Autodesk Inventor part; units mm, degrees
(part 10 of 16)
  spline S60 degree 3 poles (-53.3395, 81.2156) (-53.1853, 81.2213) (-53.0309, 81.2199) (-52.8769, 81.21) (-52.8312, 81.2071) (-52.7854, 81.2035) (-52.7398, 81.199) (-52.6969, 81.1948) (-52.6541, 81.1899) (-52.6114, 81.1843) (-52.5714, 81.179) (-52.5315, 81.1731) (-52.4918, 81.1665) (-52.4548, 81.1604) (-52.4178, 81.1536) (-52.381, 81.1462) (-52.347, 81.1394) (-52.313, 81.132) (-52.2792, 81.124) (-52.2481, 81.1167) (-52.2171, 81.1088) (-52.1863, 81.1004) (-52.1581, 81.0928) (-52.13, 81.0847) (-52.1022, 81.0761) (-52.0769, 81.0683) (-52.0519, 81.06) (-52.0269, 81.0515) (-52.0045, 81.0438) (-51.9821, 81.0359) (-51.9603, 81.0272) (-51.9409, 81.0196) (-51.922, 81.0114) (-51.9022, 81.0039) (-51.8655, 80.99) (-51.8262, 80.9786) (-51.7969, 80.9544) (-51.7748, 80.9361) (-51.7584, 80.9104) (-51.7398, 80.8873) (-51.7243, 80.868) (-51.7072, 80.8504) (-51.6902, 80.8327) (-51.6736, 80.8155) (-51.6571, 80.7981) (-51.6403, 80.781) (-51.6238, 80.7644) (-51.6071, 80.7481) (-51.5901, 80.7321) (-51.5735, 80.7165) (-51.5567, 80.7011) (-51.5397, 80.686) (-51.5231, 80.6713) (-51.5062, 80.6569) (-51.4891, 80.6428) (-51.4725, 80.629) (-51.4556, 80.6155) (-51.4384, 80.6023) (-51.4217, 80.5894) (-51.4048, 80.5768) (-51.3876, 80.5645) (-51.3708, 80.5525) (-51.3538, 80.5409) (-51.3366, 80.5295) (-51.3198, 80.5185) (-51.3028, 80.5077) (-51.2856, 80.4973) (-51.2687, 80.4871) (-51.2516, 80.4773) (-51.2344, 80.4678) (-51.2174, 80.4585) (-51.2003, 80.4496) (-51.183, 80.4411) (-51.166, 80.4327) (-51.1488, 80.4247) (-51.1314, 80.4171) (-51.1143, 80.4096) (-51.0969, 80.4026) (-51.0795, 80.396) (-51.0622, 80.3894) (-51.0448, 80.3833) (-51.0272, 80.3777) (-51.0097, 80.3721) (-50.9921, 80.367) (-50.9744, 80.3624) (-50.9567, 80.3578) (-50.9389, 80.3538) (-50.921, 80.3503) (-50.903, 80.3468) (-50.8849, 80.3438) (-50.8667, 80.3415) (-50.8484, 80.3392) (-50.83, 80.3375) (-50.8116, 80.3364) (-50.7929, 80.3354) (-50.7742, 80.335) (-50.7555, 80.3354) (-50.7363, 80.3358) (-50.7172, 80.3369) (-50.6982, 80.3389) (-50.6787, 80.341) (-50.6593, 80.3439) (-50.64, 80.3477) (-50.6201, 80.3516) (-50.6004, 80.3565) (-50.581, 80.3623) (-50.561, 80.3684) (-50.5413, 80.3755) (-50.522, 80.3836) (-50.502, 80.392) (-50.4825, 80.4016) (-50.4637, 80.4122) (-50.4442, 80.4232) (-50.4254, 80.4353) (-50.4075, 80.4485) (-50.3891, 80.4621) (-50.3715, 80.4769) (-50.3549, 80.4925) (-50.343, 80.5036) (-50.3316, 80.5152) (-50.3204, 80.527) (-50.2664, 80.5833) (-50.2161, 80.6432) (-50.1623, 80.6997) (-50.1085, 80.7562) (-50.0512, 80.8094) (-49.9976, 80.8661) (-49.9864, 80.878) (-49.9754, 80.8899) (-49.9649, 80.9023) (-49.9501, 80.9197) (-49.9362, 80.9379) (-49.9236, 80.957) (-49.9112, 80.9756) (-49.9001, 80.995) (-49.8901, 81.0149) (-49.8804, 81.0343) (-49.8718, 81.0542) (-49.8644, 81.0746) (-49.8572, 81.0942) (-49.8511, 81.1143) (-49.846, 81.1346) (-49.8411, 81.1543) (-49.8373, 81.1742) (-49.8343, 81.1942) (-49.8315, 81.2137) (-49.8295, 81.2332) (-49.8285, 81.2528) (-49.8274, 81.2719) (-49.8272, 81.291) (-49.8278, 81.3102) (-49.8283, 81.3289) (-49.8296, 81.3476) (-49.8316, 81.3662) (-49.8335, 81.3846) (-49.8362, 81.4028) (-49.8394, 81.421) (-49.8426, 81.439) (-49.8465, 81.4569) (-49.8508, 81.4747) (-49.8552, 81.4925) (-49.8602, 81.5101) (-49.8656, 81.5275) (-49.8711, 81.545) (-49.877, 81.5623) (-49.8835, 81.5795) (-49.8899, 81.5968) (-49.8969, 81.6139) (-49.9043, 81.6308) (-49.9118, 81.6479) (-49.9197, 81.6648) (-49.928, 81.6816) (-49.9364, 81.6986) (-49.9453, 81.7154) (-49.9545, 81.7319) (-49.9639, 81.7488) (-49.9736, 81.7655) (-49.9837, 81.7819) (-49.994, 81.7987) (-50.0047, 81.8153) (-50.0157, 81.8316) (-50.027, 81.8483) (-50.0385, 81.8648) (-50.0504, 81.881) (-50.0626, 81.8976) (-50.0751, 81.914) (-50.0879, 81.9302) (-50.101, 81.9467) (-50.1144, 81.963) (-50.1281, 81.9791) (-50.1421, 81.9956) (-50.1565, 82.0118) (-50.1711, 82.0277) (-50.186, 82.0441) (-50.2013, 82.0602) (-50.2168, 82.0761) (-50.2327, 82.0924) (-50.2489, 82.1084) (-50.2653, 82.1241) (-50.2821, 82.1403) (-50.2992, 82.1563) (-50.3166, 82.1718) (-50.3345, 82.1878) (-50.3527, 82.2035) (-50.3707, 82.2192) (-50.3893, 82.2353) (-50.4076, 82.2515) (-50.4277, 82.266) (-50.4517, 82.2834) (-50.4782, 82.2985) (-50.4976, 82.3197) (-50.5232, 82.3477) (-50.5364, 82.3865) (-50.5522, 82.4225) (-50.5606, 82.4418) (-50.5698, 82.4603) (-50.5784, 82.4793) (-50.5881, 82.5007) (-50.5971, 82.5226) (-50.6059, 82.5446) (-50.6157, 82.5691) (-50.6251, 82.5938) (-50.6342, 82.6186) (-50.6441, 82.646) (-50.6536, 82.6736) (-50.6627, 82.7014) (-50.6726, 82.7318) (-50.6819, 82.7623) (-50.6908, 82.793) (-50.7005, 82.8264) (-50.7095, 82.86) (-50.718, 82.8936) (-50.7272, 82.93) (-50.7358, 82.9666) (-50.7438, 83.0032) (-50.7523, 83.0426) (-50.7602, 83.0822) (-50.7674, 83.1218) (-50.7752, 83.1642) (-50.7822, 83.2067) (-50.7885, 83.2493) (-50.7952, 83.2947) (-50.8011, 83.3402) (-50.8063, 83.3858) (-50.8237, 83.539) (-50.8328, 83.6932) (-50.8347, 83.8475) knots 0 0 0 0 0.065113 0.065113 0.065113 0.084473 0.084473 0.084473 0.102659 0.102659 0.102659 0.119672 0.119672 0.119672 0.135512 0.135512 0.135512 0.150178 0.150178 0.150178 0.163672 0.163672 0.163672 0.175991 0.175991 0.175991 0.187138 0.187138 0.187138 0.197111 0.197111 0.197111 0.205911 0.205911 0.205911 0.222284 0.222284 0.222284 0.234681 0.234681 0.234681 0.24506 0.24506 0.24506 0.255176 0.255176 0.255176 0.265035 0.265035 0.265035 0.274643 0.274643 0.274643 0.284008 0.284008 0.284008 0.293139 0.293139 0.293139 0.302047 0.302047 0.302047 0.310743 0.310743 0.310743 0.319241 0.319241 0.319241 0.327556 0.327556 0.327556 0.335706 0.335706 0.335706 0.343713 0.343713 0.343713 0.351599 0.351599 0.351599 0.359392 0.359392 0.359392 0.367126 0.367126 0.367126 0.374835 0.374835 0.374835 0.382562 0.382562 0.382562 0.390352 0.390352 0.390352 0.398256 0.398256 0.398256 0.406325 0.406325 0.406325 0.41461 0.41461 0.41461 0.423156 0.423156 0.423156 0.431994 0.431994 0.431994 0.441132 0.441132 0.441132 0.450548 0.450548 0.450548 0.460189 0.460189 0.460189 0.467051 0.467051 0.467051 0.5 0.5 0.5 0.532949 0.532949 0.532949 0.539811 0.539811 0.539811 0.549452 0.549452 0.549452 0.558868 0.558868 0.558868 0.568006 0.568006 0.568006 0.576844 0.576844 0.576844 0.58539 0.58539 0.58539 0.593675 0.593675 0.593675 0.601744 0.601744 0.601744 0.609648 0.609648 0.609648 0.617438 0.617438 0.617438 0.625165 0.625165 0.625165 0.632874 0.632874 0.632874 0.640608 0.640608 0.640608 0.648401 0.648401 0.648401 0.656287 0.656287 0.656287 0.664294 0.664294 0.664294 0.672444 0.672444 0.672444 0.680759 0.680759 0.680759 0.689257 0.689257 0.689257 0.697953 0.697953 0.697953 0.706861 0.706861 0.706861 0.715992 0.715992 0.715992 0.725357 0.725357 0.725357 0.734965 0.734965 0.734965 0.744824 0.744824 0.744824 0.75494 0.75494 0.75494 0.765319 0.765319 0.765319 0.777716 0.777716 0.777716 0.794089 0.794089 0.794089 0.802889 0.802889 0.802889 0.812862 0.812862 0.812862 0.824009 0.824009 0.824009 0.836328 0.836328 0.836328 0.849822 0.849822 0.849822 0.864488 0.864488 0.864488 0.880328 0.880328 0.880328 0.897341 0.897341 0.897341 0.915527 0.915527 0.915527 0.934887 0.934887 0.934887 1 1 1 1
  arc A262 (-53.3395, 81.2156) -> (-53.8156, 80.3417) centre (-45.7832, 76.5321) ccw
  spline S61 degree 3 poles (-54.6689, 76.81) (-54.5382, 76.892) (-54.4037, 76.968) (-54.2655, 77.0365) (-54.2244, 77.0568) (-54.183, 77.0765) (-54.1412, 77.0955) (-54.102, 77.1133) (-54.0625, 77.1305) (-54.0227, 77.147) (-53.9854, 77.1624) (-53.9479, 77.1772) (-53.9102, 77.1914) (-53.8751, 77.2045) (-53.8397, 77.2172) (-53.8041, 77.2291) (-53.7712, 77.2403) (-53.7381, 77.2508) (-53.7048, 77.2608) (-53.6742, 77.27) (-53.6435, 77.2787) (-53.6126, 77.2869) (-53.5843, 77.2943) (-53.556, 77.3014) (-53.5275, 77.3078) (-53.5018, 77.3137) (-53.476, 77.3191) (-53.45, 77.3242) (-53.4268, 77.3287) (-53.4035, 77.333) (-53.3802, 77.3365) (-53.3597, 77.3395) (-53.3391, 77.3419) (-53.3183, 77.3453) (-53.2796, 77.3516) (-53.2398, 77.3614) (-53.2024, 77.3551) (-53.174, 77.3503) (-53.147, 77.3363) (-53.1194, 77.3255) (-53.0962, 77.3165) (-53.0727, 77.3099) (-53.0491, 77.3031) (-53.0261, 77.2964) (-53.0031, 77.2896) (-52.98, 77.2832) (-52.9575, 77.2771) (-52.9348, 77.2714) (-52.9121, 77.266) (-52.89, 77.2608) (-52.8677, 77.2558) (-52.8454, 77.2513) (-52.8237, 77.2468) (-52.8019, 77.2428) (-52.78, 77.2391) (-52.7587, 77.2355) (-52.7373, 77.2322) (-52.7158, 77.2294) (-52.6949, 77.2266) (-52.6739, 77.2241) (-52.6529, 77.2221) (-52.6324, 77.2201) (-52.6119, 77.2185) (-52.5913, 77.2173) (-52.5712, 77.2161) (-52.5511, 77.2153) (-52.531, 77.2149) (-52.5113, 77.2145) (-52.4916, 77.2145) (-52.4719, 77.215) (-52.4526, 77.2154) (-52.4333, 77.2162) (-52.414, 77.2175) (-52.3951, 77.2187) (-52.3762, 77.2204) (-52.3573, 77.2225) (-52.3388, 77.2246) (-52.3203, 77.2272) (-52.3018, 77.2302) (-52.2836, 77.2331) (-52.2654, 77.2366) (-52.2474, 77.2405) (-52.2295, 77.2444) (-52.2117, 77.2488) (-52.194, 77.2537) (-52.1764, 77.2586) (-52.159, 77.2639) (-52.1417, 77.2699) (-52.1244, 77.2758) (-52.1073, 77.2823) (-52.0904, 77.2894) (-52.0733, 77.2965) (-52.0566, 77.3042) (-52.0401, 77.3126) (-52.0234, 77.321) (-52.007, 77.33) (-51.9909, 77.3397) (-51.9746, 77.3496) (-51.9586, 77.3602) (-51.9431, 77.3714) (-51.9272, 77.3829) (-51.9119, 77.3952) (-51.8971, 77.4081) (-51.8818, 77.4214) (-51.8672, 77.4355) (-51.8533, 77.4503) (-51.839, 77.4655) (-51.8255, 77.4815) (-51.8128, 77.4982) (-51.7998, 77.5155) (-51.7877, 77.5335) (-51.7767, 77.5522) (-51.7653, 77.5714) (-51.7551, 77.5913) (-51.7461, 77.6117) (-51.737, 77.6327) (-51.7292, 77.6542) (-51.7226, 77.6761) (-51.7179, 77.6916) (-51.7138, 77.7074) (-51.7099, 77.7232) (-51.6913, 77.799) (-51.6777, 77.876) (-51.6594, 77.9518) (-51.641, 78.0277) (-51.618, 78.1024) (-51.6, 78.1783) (-51.5962, 78.1941) (-51.5927, 78.21) (-51.5897, 78.226) (-51.5856, 78.2485) (-51.5827, 78.2712) (-51.5813, 78.294) (-51.5799, 78.3163) (-51.5799, 78.3386) (-51.5813, 78.3609) (-51.5826, 78.3825) (-51.5851, 78.4041) (-51.5888, 78.4254) (-51.5924, 78.446) (-51.5972, 78.4665) (-51.603, 78.4866) (-51.6086, 78.5061) (-51.6151, 78.5253) (-51.6226, 78.5441) (-51.6299, 78.5623) (-51.638, 78.5802) (-51.6469, 78.5977) (-51.6555, 78.6148) (-51.6649, 78.6315) (-51.6749, 78.6478) (-51.6847, 78.6637) (-51.6952, 78.6792) (-51.7062, 78.6944) (-51.7171, 78.7093) (-51.7285, 78.7238) (-51.7404, 78.7379) (-51.7522, 78.7519) (-51.7645, 78.7655) (-51.7772, 78.7787) (-51.7898, 78.7919) (-51.8029, 78.8047) (-51.8163, 78.8171) (-51.8298, 78.8295) (-51.8436, 78.8415) (-51.8578, 78.8531) (-51.8721, 78.8649) (-51.8866, 78.8762) (-51.9015, 78.8872) (-51.9165, 78.8983) (-51.9318, 78.909) (-51.9474, 78.9193) (-51.9632, 78.9298) (-51.9793, 78.9399) (-51.9955, 78.9497) (-52.0121, 78.9596) (-52.0289, 78.9691) (-52.0459, 78.9783) (-52.0632, 78.9877) (-52.0807, 78.9967) (-52.0984, 79.0054) (-52.1165, 79.0142) (-52.1348, 79.0227) (-52.1532, 79.0308) (-52.172, 79.0391) (-52.191, 79.0471) (-52.2102, 79.0546) (-52.2298, 79.0624) (-52.2496, 79.0698) (-52.2695, 79.0769) (-52.2899, 79.0841) (-52.3104, 79.091) (-52.331, 79.0975) (-52.3521, 79.1042) (-52.3734, 79.1106) (-52.3948, 79.1166) (-52.4167, 79.1227) (-52.4387, 79.1285) (-52.4608, 79.1339) (-52.4835, 79.1395) (-52.5062, 79.1448) (-52.5291, 79.1496) (-52.5526, 79.1545) (-52.5762, 79.1589) (-52.5996, 79.1635) (-52.6237, 79.1682) (-52.6477, 79.173) (-52.6724, 79.1756) (-52.7019, 79.1787) (-52.7323, 79.1785) (-52.7597, 79.1872) (-52.7959, 79.1986) (-52.8268, 79.2255) (-52.8584, 79.2488) (-52.8754, 79.2614) (-52.8926, 79.2728) (-52.9095, 79.2849) (-52.9286, 79.2986) (-52.9474, 79.3131) (-52.966, 79.3277) (-52.9867, 79.3441) (-53.0072, 79.3607) (-53.0275, 79.3777) (-53.0498, 79.3964) (-53.0718, 79.4156) (-53.0935, 79.4351) (-53.1173, 79.4565) (-53.1407, 79.4783) (-53.1638, 79.5004) (-53.1888, 79.5245) (-53.2134, 79.5491) (-53.2376, 79.574) (-53.2638, 79.6009) (-53.2895, 79.6282) (-53.3147, 79.656) (-53.3418, 79.6858) (-53.3684, 79.7161) (-53.3945, 79.7468) (-53.4224, 79.7797) (-53.4497, 79.813) (-53.4765, 79.8468) (-53.505, 79.8827) (-53.5329, 79.9191) (-53.5601, 79.956) (-53.6519, 80.08) (-53.7368, 80.2091) (-53.8156, 80.3417) knots 0 0 0 0 0.065113 0.065113 0.065113 0.084473 0.084473 0.084473 0.102659 0.102659 0.102659 0.119672 0.119672 0.119672 0.135512 0.135512 0.135512 0.150178 0.150178 0.150178 0.163672 0.163672 0.163672 0.175991 0.175991 0.175991 0.187138 0.187138 0.187138 0.197111 0.197111 0.197111 0.205911 0.205911 0.205911 0.222284 0.222284 0.222284 0.234681 0.234681 0.234681 0.24506 0.24506 0.24506 0.255176 0.255176 0.255176 0.265035 0.265035 0.265035 0.274643 0.274643 0.274643 0.284008 0.284008 0.284008 0.293139 0.293139 0.293139 0.302047 0.302047 0.302047 0.310743 0.310743 0.310743 0.319241 0.319241 0.319241 0.327556 0.327556 0.327556 0.335706 0.335706 0.335706 0.343713 0.343713 0.343713 0.351599 0.351599 0.351599 0.359392 0.359392 0.359392 0.367126 0.367126 0.367126 0.374835 0.374835 0.374835 0.382562 0.382562 0.382562 0.390352 0.390352 0.390352 0.398256 0.398256 0.398256 0.406325 0.406325 0.406325 0.41461 0.41461 0.41461 0.423156 0.423156 0.423156 0.431994 0.431994 0.431994 0.441132 0.441132 0.441132 0.450548 0.450548 0.450548 0.460189 0.460189 0.460189 0.467051 0.467051 0.467051 0.5 0.5 0.5 0.532949 0.532949 0.532949 0.539811 0.539811 0.539811 0.549452 0.549452 0.549452 0.558868 0.558868 0.558868 0.568006 0.568006 0.568006 0.576844 0.576844 0.576844 0.58539 0.58539 0.58539 0.593675 0.593675 0.593675 0.601744 0.601744 0.601744 0.609648 0.609648 0.609648 0.617438 0.617438 0.617438 0.625165 0.625165 0.625165 0.632874 0.632874 0.632874 0.640608 0.640608 0.640608 0.648401 0.648401 0.648401 0.656287 0.656287 0.656287 0.664294 0.664294 0.664294 0.672444 0.672444 0.672444 0.680759 0.680759 0.680759 0.689257 0.689257 0.689257 0.697953 0.697953 0.697953 0.706861 0.706861 0.706861 0.715992 0.715992 0.715992 0.725357 0.725357 0.725357 0.734965 0.734965 0.734965 0.744824 0.744824 0.744824 0.75494 0.75494 0.75494 0.765319 0.765319 0.765319 0.777716 0.777716 0.777716 0.794089 0.794089 0.794089 0.802889 0.802889 0.802889 0.812862 0.812862 0.812862 0.824009 0.824009 0.824009 0.836328 0.836328 0.836328 0.849822 0.849822 0.849822 0.864488 0.864488 0.864488 0.880328 0.880328 0.880328 0.897341 0.897341 0.897341 0.915527 0.915527 0.915527 0.934887 0.934887 0.934887 1 1 1 1
  arc A263 (-54.6689, 76.81) -> (-54.6443, 75.8151) centre (-45.7832, 76.5321) ccw
  spline S62 degree 3 poles (-53.6173, 72.3299) (-53.5452, 72.4663) (-53.4667, 72.5994) (-53.3813, 72.7278) (-53.3558, 72.7659) (-53.3298, 72.8037) (-53.3031, 72.841) (-53.2781, 72.8761) (-53.2524, 72.9107) (-53.2262, 72.9449) (-53.2016, 72.9768) (-53.1766, 73.0084) (-53.151, 73.0396) (-53.1271, 73.0685) (-53.1028, 73.0971) (-53.078, 73.1253) (-53.0551, 73.1514) (-53.0317, 73.1771) (-53.0079, 73.2024) (-52.986, 73.2257) (-52.9637, 73.2486) (-52.941, 73.2711) (-52.9203, 73.2917) (-52.8992, 73.3119) (-52.8778, 73.3317) (-52.8585, 73.3497) (-52.8388, 73.3673) (-52.8189, 73.3847) (-52.8011, 73.4002) (-52.783, 73.4156) (-52.7646, 73.4302) (-52.7483, 73.4431) (-52.7317, 73.4554) (-52.7154, 73.4688) (-52.6849, 73.4936) (-52.6555, 73.522) (-52.6199, 73.5353) (-52.5929, 73.5453) (-52.5625, 73.5466) (-52.5332, 73.5512) (-52.5087, 73.5549) (-52.485, 73.561) (-52.4611, 73.5668) (-52.4379, 73.5726) (-52.4146, 73.5781) (-52.3914, 73.5842) (-52.3688, 73.5901) (-52.3463, 73.5965) (-52.3239, 73.6032) (-52.3021, 73.6098) (-52.2804, 73.6166) (-52.2588, 73.6238) (-52.2378, 73.6309) (-52.2169, 73.6382) (-52.1961, 73.646) (-52.1758, 73.6535) (-52.1556, 73.6614) (-52.1356, 73.6696) (-52.1161, 73.6777) (-52.0968, 73.6861) (-52.0775, 73.6948) (-52.0588, 73.7033) (-52.0402, 73.7122) (-52.0218, 73.7214) (-52.0038, 73.7305) (-51.986, 73.7398) (-51.9683, 73.7496) (-51.9511, 73.7591) (-51.934, 73.7689) (-51.9172, 73.7792) (-51.9007, 73.7892) (-51.8844, 73.7995) (-51.8683, 73.8103) (-51.8526, 73.8208) (-51.837, 73.8317) (-51.8218, 73.843) (-51.8067, 73.8541) (-51.792, 73.8655) (-51.7775, 73.8774) (-51.7632, 73.889) (-51.7492, 73.9011) (-51.7355, 73.9135) (-51.722, 73.9258) (-51.7088, 73.9385) (-51.6959, 73.9516) (-51.6831, 73.9646) (-51.6707, 73.978) (-51.6587, 73.9918) (-51.6467, 74.0056) (-51.6351, 74.0198) (-51.624, 74.0344) (-51.6128, 74.0491) (-51.6021, 74.0641) (-51.592, 74.0796) (-51.5818, 74.0952) (-51.5721, 74.1113) (-51.563, 74.1277) (-51.5538, 74.1444) (-51.5453, 74.1616) (-51.5375, 74.179) (-51.5295, 74.197) (-51.5223, 74.2152) (-51.5159, 74.2338) (-51.5094, 74.253) (-51.5038, 74.2725) (-51.4992, 74.2922) (-51.4944, 74.3126) (-51.4907, 74.3332) (-51.4881, 74.354) (-51.4854, 74.3755) (-51.4839, 74.3971) (-51.4837, 74.4188) (-51.4835, 74.4411) (-51.4845, 74.4635) (-51.487, 74.4856) (-51.4896, 74.5084) (-51.4936, 74.5309) (-51.4988, 74.5531) (-51.5025, 74.569) (-51.5069, 74.5846) (-51.5114, 74.6002) (-51.5332, 74.6752) (-51.5599, 74.7487) (-51.5819, 74.8235) (-51.604, 74.8984) (-51.6214, 74.9746) (-51.6438, 75.0494) (-51.6484, 75.065) (-51.6533, 75.0805) (-51.6587, 75.0958) (-51.6664, 75.1173) (-51.6752, 75.1385) (-51.6854, 75.1589) (-51.6954, 75.1789) (-51.7066, 75.1983) (-51.7189, 75.2169) (-51.7308, 75.235) (-51.7438, 75.2524) (-51.7577, 75.269) (-51.7711, 75.285) (-51.7854, 75.3003) (-51.8005, 75.3149) (-51.8151, 75.3289) (-51.8304, 75.3423) (-51.8463, 75.3548) (-51.8617, 75.367) (-51.8776, 75.3785) (-51.8941, 75.3892) (-51.9101, 75.3996) (-51.9266, 75.4094) (-51.9434, 75.4185) (-51.9599, 75.4274) (-51.9767, 75.4356) (-51.9938, 75.4432) (-52.0107, 75.4507) (-52.0278, 75.4575) (-52.0452, 75.4638) (-52.0624, 75.47) (-52.0798, 75.4757) (-52.0974, 75.4808) (-52.115, 75.4858) (-52.1327, 75.4904) (-52.1505, 75.4944) (-52.1684, 75.4984) (-52.1864, 75.5019) (-52.2044, 75.5049) (-52.2227, 75.5079) (-52.241, 75.5104) (-52.2593, 75.5125) (-52.2779, 75.5146) (-52.2965, 75.5162) (-52.3151, 75.5174) (-52.3341, 75.5186) (-52.353, 75.5193) (-52.372, 75.5196) (-52.3913, 75.5199) (-52.4106, 75.5198) (-52.4299, 75.5193) (-52.4496, 75.5188) (-52.4693, 75.5178) (-52.4889, 75.5164) (-52.509, 75.515) (-52.5291, 75.5132) (-52.5491, 75.5111) (-52.5696, 75.5088) (-52.59, 75.5062) (-52.6104, 75.5032) (-52.6313, 75.5001) (-52.6521, 75.4967) (-52.6729, 75.4928) (-52.6941, 75.4889) (-52.7153, 75.4846) (-52.7365, 75.48) (-52.7581, 75.4752) (-52.7797, 75.47) (-52.8012, 75.4645) (-52.8233, 75.4589) (-52.8452, 75.4529) (-52.8671, 75.4466) (-52.8895, 75.4401) (-52.9118, 75.4332) (-52.934, 75.426) (-52.9568, 75.4185) (-52.9795, 75.4105) (-53.0021, 75.4027) (-53.0253, 75.3947) (-53.0485, 75.3869) (-53.0711, 75.3768) (-53.0982, 75.3648) (-53.1245, 75.3494) (-53.1526, 75.3432) (-53.1897, 75.335) (-53.2298, 75.3429) (-53.2689, 75.3473) (-53.2898, 75.3496) (-53.3105, 75.351) (-53.3311, 75.353) (-53.3546, 75.3553) (-53.3781, 75.3584) (-53.4015, 75.3618) (-53.4276, 75.3656) (-53.4537, 75.3697) (-53.4797, 75.3743) (-53.5084, 75.3794) (-53.5371, 75.385) (-53.5656, 75.391) (-53.5969, 75.3977) (-53.6281, 75.4048) (-53.6591, 75.4125) (-53.6928, 75.4208) (-53.7264, 75.4298) (-53.7599, 75.4392) (-53.796, 75.4494) (-53.8319, 75.4603) (-53.8676, 75.4717) (-53.906, 75.484) (-53.9442, 75.4969) (-53.9822, 75.5105) (-54.0227, 75.525) (-54.063, 75.5402) (-54.1031, 75.5561) (-54.1458, 75.5729) (-54.1881, 75.5905) (-54.2302, 75.6088) (-54.3716, 75.6704) (-54.5097, 75.7397) (-54.6443, 75.8151) knots 0 0 0 0 0.065113 0.065113 0.065113 0.084473 0.084473 0.084473 0.102659 0.102659 0.102659 0.119672 0.119672 0.119672 0.135512 0.135512 0.135512 0.150178 0.150178 0.150178 0.163672 0.163672 0.163672 0.175991 0.175991 0.175991 0.187138 0.187138 0.187138 0.197111 0.197111 0.197111 0.205911 0.205911 0.205911 0.222284 0.222284 0.222284 0.234681 0.234681 0.234681 0.24506 0.24506 0.24506 0.255176 0.255176 0.255176 0.265035 0.265035 0.265035 0.274643 0.274643 0.274643 0.284008 0.284008 0.284008 0.293139 0.293139 0.293139 0.302047 0.302047 0.302047 0.310743 0.310743 0.310743 0.319241 0.319241 0.319241 0.327556 0.327556 0.327556 0.335706 0.335706 0.335706 0.343713 0.343713 0.343713 0.351599 0.351599 0.351599 0.359392 0.359392 0.359392 0.367126 0.367126 0.367126 0.374835 0.374835 0.374835 0.382562 0.382562 0.382562 0.390352 0.390352 0.390352 0.398256 0.398256 0.398256 0.406325 0.406325 0.406325 0.41461 0.41461 0.41461 0.423156 0.423156 0.423156 0.431994 0.431994 0.431994 0.441132 0.441132 0.441132 0.450548 0.450548 0.450548 0.460189 0.460189 0.460189 0.467051 0.467051 0.467051 0.5 0.5 0.5 0.532949 0.532949 0.532949 0.539811 0.539811 0.539811 0.549452 0.549452 0.549452 0.558868 0.558868 0.558868 0.568006 0.568006 0.568006 0.576844 0.576844 0.576844 0.58539 0.58539 0.58539 0.593675 0.593675 0.593675 0.601744 0.601744 0.601744 0.609648 0.609648 0.609648 0.617438 0.617438 0.617438 0.625165 0.625165 0.625165 0.632874 0.632874 0.632874 0.640608 0.640608 0.640608 0.648401 0.648401 0.648401 0.656287 0.656287 0.656287 0.664294 0.664294 0.664294 0.672444 0.672444 0.672444 0.680759 0.680759 0.680759 0.689257 0.689257 0.689257 0.697953 0.697953 0.697953 0.706861 0.706861 0.706861 0.715992 0.715992 0.715992 0.725357 0.725357 0.725357 0.734965 0.734965 0.734965 0.744824 0.744824 0.744824 0.75494 0.75494 0.75494 0.765319 0.765319 0.765319 0.777716 0.777716 0.777716 0.794089 0.794089 0.794089 0.802889 0.802889 0.802889 0.812862 0.812862 0.812862 0.824009 0.824009 0.824009 0.836328 0.836328 0.836328 0.849822 0.849822 0.849822 0.864488 0.864488 0.864488 0.880328 0.880328 0.880328 0.897341 0.897341 0.897341 0.915527 0.915527 0.915527 0.934887 0.934887 0.934887 1 1 1 1
  arc A264 (-53.6173, 72.3299) -> (-53.0986, 71.4807) centre (-45.7832, 76.5321) ccw
  spline S63 degree 3 poles (-50.4667, 68.9759) (-50.4723, 69.13) (-50.471, 69.2845) (-50.4611, 69.4384) (-50.4582, 69.4842) (-50.4545, 69.5299) (-50.4501, 69.5756) (-50.4459, 69.6185) (-50.441, 69.6613) (-50.4354, 69.704) (-50.4301, 69.744) (-50.4242, 69.7838) (-50.4176, 69.8236) (-50.4114, 69.8606) (-50.4047, 69.8975) (-50.3973, 69.9343) (-50.3905, 69.9684) (-50.3831, 70.0023) (-50.3751, 70.0362) (-50.3677, 70.0673) (-50.3599, 70.0983) (-50.3515, 70.1291) (-50.3439, 70.1573) (-50.3358, 70.1853) (-50.3271, 70.2132) (-50.3193, 70.2384) (-50.3111, 70.2635) (-50.3026, 70.2885) (-50.2949, 70.3109) (-50.287, 70.3332) (-50.2783, 70.3551) (-50.2707, 70.3744) (-50.2624, 70.3934) (-50.2549, 70.4131) (-50.241, 70.4498) (-50.2297, 70.4892) (-50.2055, 70.5185) (-50.1872, 70.5406) (-50.1615, 70.557) (-50.1384, 70.5755) (-50.119, 70.5911) (-50.1015, 70.6082) (-50.0838, 70.6252) (-50.0666, 70.6417) (-50.0491, 70.6582) (-50.0321, 70.6751) (-50.0155, 70.6915) (-49.9992, 70.7083) (-49.9832, 70.7253) (-49.9676, 70.7418) (-49.9522, 70.7586) (-49.9371, 70.7757) (-49.9224, 70.7923) (-49.908, 70.8091) (-49.8938, 70.8262) (-49.88, 70.8429) (-49.8665, 70.8598) (-49.8533, 70.8769) (-49.8405, 70.8937) (-49.8279, 70.9106) (-49.8156, 70.9278) (-49.8036, 70.9445) (-49.792, 70.9615) (-49.7806, 70.9787) (-49.7695, 70.9955) (-49.7588, 71.0126) (-49.7484, 71.0298) (-49.7382, 71.0467) (-49.7284, 71.0637) (-49.7189, 71.081) (-49.7096, 71.0979) (-49.7007, 71.1151) (-49.6922, 71.1324) (-49.6838, 71.1494) (-49.6758, 71.1666) (-49.6682, 71.184) (-49.6607, 71.2011) (-49.6537, 71.2184) (-49.647, 71.2359) (-49.6405, 71.2532) (-49.6344, 71.2706) (-49.6288, 71.2882) (-49.6232, 71.3056) (-49.6181, 71.3232) (-49.6135, 71.341) (-49.6089, 71.3587) (-49.6049, 71.3765) (-49.6014, 71.3944) (-49.5979, 71.4124) (-49.5949, 71.4305) (-49.5926, 71.4486) (-49.5903, 71.4669) (-49.5885, 71.4853) (-49.5875, 71.5037) (-49.5864, 71.5224) (-49.5861, 71.5412) (-49.5865, 71.5599) (-49.5869, 71.579) (-49.588, 71.5981) (-49.59, 71.6171) (-49.592, 71.6367) (-49.5949, 71.6561) (-49.5987, 71.6754) (-49.6027, 71.6952) (-49.6075, 71.7149) (-49.6134, 71.7343) (-49.6194, 71.7544) (-49.6265, 71.7741) (-49.6347, 71.7934) (-49.6431, 71.8133) (-49.6527, 71.8328) (-49.6633, 71.8517) (-49.6743, 71.8711) (-49.6864, 71.8899) (-49.6996, 71.9079) (-49.7132, 71.9263) (-49.7279, 71.9438) (-49.7436, 71.9605) (-49.7547, 71.9723) (-49.7663, 71.9837) (-49.778, 71.995) (-49.8344, 72.049) (-49.8942, 72.0993) (-49.9508, 72.1531) (-50.0073, 72.2069) (-50.0605, 72.2642) (-50.1172, 72.3178) (-50.129, 72.3289) (-50.141, 72.34) (-50.1534, 72.3505) (-50.1708, 72.3653) (-50.189, 72.3792) (-50.2081, 72.3918) (-50.2267, 72.4041) (-50.246, 72.4153) (-50.266, 72.4253) (-50.2854, 72.435) (-50.3053, 72.4435) (-50.3256, 72.451) (-50.3453, 72.4582) (-50.3654, 72.4643) (-50.3857, 72.4693) (-50.4054, 72.4742) (-50.4253, 72.4781) (-50.4453, 72.481) (-50.4647, 72.4839) (-50.4843, 72.4858) (-50.5039, 72.4869) (-50.523, 72.4879) (-50.5421, 72.4881) (-50.5612, 72.4876) (-50.58, 72.487) (-50.5987, 72.4858) (-50.6173, 72.4838) (-50.6356, 72.4818) (-50.6539, 72.4792) (-50.6721, 72.476) (-50.6901, 72.4727) (-50.708, 72.4689) (-50.7258, 72.4645) (-50.7435, 72.4601) (-50.7611, 72.4552) (-50.7786, 72.4498) (-50.7961, 72.4443) (-50.8134, 72.4383) (-50.8305, 72.4319) (-50.8478, 72.4254) (-50.8649, 72.4185) (-50.8819, 72.4111) (-50.899, 72.4036) (-50.9159, 72.3957) (-50.9327, 72.3874) (-50.9496, 72.3789) (-50.9664, 72.3701) (-50.983, 72.3609) (-50.9999, 72.3515) (-51.0166, 72.3417) (-51.033, 72.3316) (-51.0498, 72.3213) (-51.0663, 72.3107) (-51.0827, 72.2996) (-51.0994, 72.2884) (-51.1159, 72.2768) (-51.1321, 72.2649) (-51.1487, 72.2528) (-51.1651, 72.2403) (-51.1813, 72.2275) (-51.1978, 72.2144) (-51.2141, 72.201) (-51.2302, 72.1873) (-51.2466, 72.1732) (-51.2628, 72.1589) (-51.2788, 72.1443) (-51.2952, 72.1293) (-51.3113, 72.1141) (-51.3272, 72.0986) (-51.3434, 72.0827) (-51.3595, 72.0665) (-51.3752, 72.0501) (-51.3914, 72.0332) (-51.4073, 72.0162) (-51.4229, 71.9988) (-51.4389, 71.9809) (-51.4545, 71.9627) (-51.4702, 71.9446) (-51.4863, 71.9261) (-51.5025, 71.9077) (-51.5171, 71.8877) (-51.5345, 71.8637) (-51.5496, 71.8372) (-51.5708, 71.8178) (-51.5988, 71.7922) (-51.6376, 71.7789) (-51.6736, 71.7632) (-51.6929, 71.7548) (-51.7114, 71.7456) (-51.7303, 71.737) (-51.7518, 71.7273) (-51.7737, 71.7182) (-51.7957, 71.7095) (-51.8202, 71.6997) (-51.8449, 71.6902) (-51.8697, 71.6812) (-51.8971, 71.6712) (-51.9247, 71.6617) (-51.9524, 71.6527) (-51.9828, 71.6428) (-52.0134, 71.6334) (-52.0441, 71.6246) (-52.0775, 71.6149) (-52.111, 71.6059) (-52.1447, 71.5973) (-52.1811, 71.5881) (-52.2176, 71.5796) (-52.2543, 71.5716) (-52.2937, 71.563) (-52.3332, 71.5552) (-52.3729, 71.5479) (-52.4153, 71.5402) (-52.4578, 71.5332) (-52.5004, 71.5269) (-52.5458, 71.5202) (-52.5913, 71.5142) (-52.6368, 71.5091) (-52.7901, 71.4916) (-52.9443, 71.4826) (-53.0986, 71.4807) knots 0 0 0 0 0.065113 0.065113 0.065113 0.084473 0.084473 0.084473 0.102659 0.102659 0.102659 0.119672 0.119672 0.119672 0.135512 0.135512 0.135512 0.150178 0.150178 0.150178 0.163672 0.163672 0.163672 0.175991 0.175991 0.175991 0.187138 0.187138 0.187138 0.197111 0.197111 0.197111 0.205911 0.205911 0.205911 0.222284 0.222284 0.222284 0.234681 0.234681 0.234681 0.24506 0.24506 0.24506 0.255176 0.255176 0.255176 0.265035 0.265035 0.265035 0.274643 0.274643 0.274643 0.284008 0.284008 0.284008 0.293139 0.293139 0.293139 0.302047 0.302047 0.302047 0.310743 0.310743 0.310743 0.319241 0.319241 0.319241 0.327556 0.327556 0.327556 0.335706 0.335706 0.335706 0.343713 0.343713 0.343713 0.351599 0.351599 0.351599 0.359392 0.359392 0.359392 0.367126 0.367126 0.367126 0.374835 0.374835 0.374835 0.382562 0.382562 0.382562 0.390352 0.390352 0.390352 0.398256 0.398256 0.398256 0.406325 0.406325 0.406325 0.41461 0.41461 0.41461 0.423156 0.423156 0.423156 0.431994 0.431994 0.431994 0.441132 0.441132 0.441132 0.450548 0.450548 0.450548 0.460189 0.460189 0.460189 0.467051 0.467051 0.467051 0.5 0.5 0.5 0.532949 0.532949 0.532949 0.539811 0.539811 0.539811 0.549452 0.549452 0.549452 0.558868 0.558868 0.558868 0.568006 0.568006 0.568006 0.576844 0.576844 0.576844 0.58539 0.58539 0.58539 0.593675 0.593675 0.593675 0.601744 0.601744 0.601744 0.609648 0.609648 0.609648 0.617438 0.617438 0.617438 0.625165 0.625165 0.625165 0.632874 0.632874 0.632874 0.640608 0.640608 0.640608 0.648401 0.648401 0.648401 0.656287 0.656287 0.656287 0.664294 0.664294 0.664294 0.672444 0.672444 0.672444 0.680759 0.680759 0.680759 0.689257 0.689257 0.689257 0.697953 0.697953 0.697953 0.706861 0.706861 0.706861 0.715992 0.715992 0.715992 0.725357 0.725357 0.725357 0.734965 0.734965 0.734965 0.744824 0.744824 0.744824 0.75494 0.75494 0.75494 0.765319 0.765319 0.765319 0.777716 0.777716 0.777716 0.794089 0.794089 0.794089 0.802889 0.802889 0.802889 0.812862 0.812862 0.812862 0.824009 0.824009 0.824009 0.836328 0.836328 0.836328 0.849822 0.849822 0.849822 0.864488 0.864488 0.864488 0.880328 0.880328 0.880328 0.897341 0.897341 0.897341 0.915527 0.915527 0.915527 0.934887 0.934887 0.934887 1 1 1 1
  arc A265 (-50.4667, 68.9759) -> (-49.5928, 68.4997) centre (-45.7832, 76.5321) ccw
  spline S64 degree 3 poles (-46.061, 67.6465) (-46.1431, 67.7772) (-46.2191, 67.9116) (-46.2876, 68.0499) (-46.3079, 68.091) (-46.3276, 68.1324) (-46.3466, 68.1742) (-46.3644, 68.2134) (-46.3815, 68.2529) (-46.398, 68.2927) (-46.4135, 68.33) (-46.4283, 68.3674) (-46.4424, 68.4052) (-46.4556, 68.4403) (-46.4682, 68.4757) (-46.4802, 68.5112) (-46.4913, 68.5441) (-46.5019, 68.5772) (-46.5119, 68.6105) (-46.5211, 68.6411) (-46.5298, 68.6719) (-46.538, 68.7028) (-46.5454, 68.731) (-46.5524, 68.7594) (-46.5589, 68.7878) (-46.5648, 68.8136) (-46.5702, 68.8394) (-46.5753, 68.8653) (-46.5798, 68.8885) (-46.5841, 68.9118) (-46.5876, 68.9351) (-46.5906, 68.9557) (-46.593, 68.9762) (-46.5963, 68.9971) (-46.6026, 69.0358) (-46.6125, 69.0756) (-46.6062, 69.113) (-46.6014, 69.1413) (-46.5873, 69.1684) (-46.5766, 69.196) (-46.5676, 69.2191) (-46.561, 69.2427) (-46.5542, 69.2663) (-46.5475, 69.2892) (-46.5407, 69.3122) (-46.5343, 69.3354) (-46.5281, 69.3579) (-46.5224, 69.3805) (-46.5171, 69.4033) (-46.5118, 69.4254) (-46.5069, 69.4476) (-46.5024, 69.4699) (-46.4979, 69.4917) (-46.4939, 69.5135) (-46.4902, 69.5354) (-46.4866, 69.5567) (-46.4833, 69.5781) (-46.4804, 69.5995) (-46.4776, 69.6205) (-46.4752, 69.6414) (-46.4732, 69.6624) (-46.4712, 69.6829) (-46.4696, 69.7035) (-46.4684, 69.724) (-46.4672, 69.7441) (-46.4664, 69.7643) (-46.466, 69.7844) (-46.4656, 69.8041) (-46.4656, 69.8238) (-46.466, 69.8435) (-46.4665, 69.8628) (-46.4673, 69.8821) (-46.4686, 69.9013) (-46.4698, 69.9203) (-46.4715, 69.9392) (-46.4736, 69.958) (-46.4757, 69.9766) (-46.4782, 69.9951) (-46.4813, 70.0135) (-46.4842, 70.0318) (-46.4877, 70.0499) (-46.4916, 70.068) (-46.4955, 70.0859) (-46.4999, 70.1037) (-46.5047, 70.1213) (-46.5096, 70.1389) (-46.515, 70.1564) (-46.521, 70.1737) (-46.5269, 70.191) (-46.5334, 70.2081) (-46.5405, 70.225) (-46.5476, 70.242) (-46.5553, 70.2588) (-46.5636, 70.2753) (-46.5721, 70.292) (-46.5811, 70.3084) (-46.5908, 70.3244) (-46.6007, 70.3408) (-46.6113, 70.3568) (-46.6225, 70.3722) (-46.634, 70.3881) (-46.6463, 70.4035) (-46.6592, 70.4183) (-46.6725, 70.4335) (-46.6866, 70.4482) (-46.7013, 70.462) (-46.7166, 70.4764) (-46.7326, 70.4899) (-46.7493, 70.5025) (-46.7666, 70.5156) (-46.7846, 70.5277) (-46.8033, 70.5387) (-46.8225, 70.5501) (-46.8424, 70.5603) (-46.8628, 70.5692) (-46.8837, 70.5784) (-46.9053, 70.5862) (-46.9272, 70.5928) (-46.9427, 70.5975) (-46.9585, 70.6016) (-46.9742, 70.6054) (-47.0501, 70.624) (-47.127, 70.6377) (-47.2029, 70.656) (-47.2787, 70.6743) (-47.3535, 70.6973) (-47.4294, 70.7154) (-47.4452, 70.7192) (-47.4611, 70.7227) (-47.4771, 70.7256) (-47.4995, 70.7298) (-47.5223, 70.7327) (-47.5451, 70.7341) (-47.5673, 70.7355) (-47.5897, 70.7354) (-47.612, 70.7341) (-47.6336, 70.7328) (-47.6552, 70.7303) (-47.6765, 70.7265) (-47.6971, 70.7229) (-47.7176, 70.7182) (-47.7377, 70.7124) (-47.7572, 70.7068) (-47.7763, 70.7002) (-47.7952, 70.6927) (-47.8134, 70.6855) (-47.8313, 70.6774) (-47.8488, 70.6685) (-47.8659, 70.6599) (-47.8826, 70.6505) (-47.8988, 70.6404) (-47.9148, 70.6306) (-47.9303, 70.6202) (-47.9455, 70.6091) (-47.9604, 70.5983) (-47.9749, 70.5868) (-47.989, 70.575) (-48.003, 70.5632) (-48.0166, 70.5509) (-48.0298, 70.5382) (-48.043, 70.5255) (-48.0557, 70.5125) (-48.0681, 70.499) (-48.0805, 70.4856) (-48.0926, 70.4717) (-48.1042, 70.4576) (-48.1159, 70.4433) (-48.1273, 70.4287) (-48.1382, 70.4139) (-48.1493, 70.3988) (-48.16, 70.3835) (-48.1704, 70.368) (-48.1809, 70.3522) (-48.191, 70.3361) (-48.2007, 70.3198) (-48.2107, 70.3033) (-48.2202, 70.2865) (-48.2294, 70.2695) (-48.2388, 70.2522) (-48.2478, 70.2347) (-48.2564, 70.217) (-48.2653, 70.1989) (-48.2738, 70.1806) (-48.2819, 70.1622) (-48.2902, 70.1433) (-48.2981, 70.1243) (-48.3057, 70.1052) (-48.3135, 70.0855) (-48.3209, 70.0658) (-48.328, 70.0459) (-48.3352, 70.0255) (-48.3421, 70.005) (-48.3486, 69.9844) (-48.3553, 69.9632) (-48.3617, 69.942) (-48.3676, 69.9206) (-48.3738, 69.8987) (-48.3795, 69.8767) (-48.385, 69.8546) (-48.3906, 69.8319) (-48.3959, 69.8091) (-48.4007, 69.7863) (-48.4056, 69.7628) (-48.41, 69.7392) (-48.4146, 69.7157) (-48.4192, 69.6916) (-48.4241, 69.6676) (-48.4267, 69.643) (-48.4297, 69.6135) (-48.4296, 69.583) (-48.4382, 69.5556) (-48.4497, 69.5194) (-48.4766, 69.4886) (-48.4999, 69.457) (-48.5124, 69.44) (-48.5239, 69.4228) (-48.536, 69.4059) (-48.5497, 69.3867) (-48.5642, 69.368) (-48.5788, 69.3494) (-48.5952, 69.3286) (-48.6118, 69.3081) (-48.6288, 69.2879) (-48.6475, 69.2655) (-48.6667, 69.2435) (-48.6862, 69.2218) (-48.7076, 69.198) (-48.7294, 69.1746) (-48.7515, 69.1516) (-48.7756, 69.1266) (-48.8001, 69.1019) (-48.825, 69.0777) (-48.8519, 69.0516) (-48.8793, 69.0259) (-48.9071, 69.0006) (-48.9369, 68.9735) (-48.9672, 68.9469) (-48.9979, 68.9208) (-49.0308, 68.893) (-49.0641, 68.8656) (-49.0978, 68.8389) (-49.1338, 68.8104) (-49.1702, 68.7825) (-49.2071, 68.7552) (-49.3311, 68.6635) (-49.4601, 68.5786) (-49.5928, 68.4997) knots 0 0 0 0 0.065113 0.065113 0.065113 0.084473 0.084473 0.084473 0.102659 0.102659 0.102659 0.119672 0.119672 0.119672 0.135512 0.135512 0.135512 0.150178 0.150178 0.150178 0.163672 0.163672 0.163672 0.175991 0.175991 0.175991 0.187138 0.187138 0.187138 0.197111 0.197111 0.197111 0.205911 0.205911 0.205911 0.222284 0.222284 0.222284 0.234681 0.234681 0.234681 0.24506 0.24506 0.24506 0.255176 0.255176 0.255176 0.265035 0.265035 0.265035 0.274643 0.274643 0.274643 0.284008 0.284008 0.284008 0.293139 0.293139 0.293139 0.302047 0.302047 0.302047 0.310743 0.310743 0.310743 0.319241 0.319241 0.319241 0.327556 0.327556 0.327556 0.335706 0.335706 0.335706 0.343713 0.343713 0.343713 0.351599 0.351599 0.351599 0.359392 0.359392 0.359392 0.367126 0.367126 0.367126 0.374835 0.374835 0.374835 0.382562 0.382562 0.382562 0.390352 0.390352 0.390352 0.398256 0.398256 0.398256 0.406325 0.406325 0.406325 0.41461 0.41461 0.41461 0.423156 0.423156 0.423156 0.431994 0.431994 0.431994 0.441132 0.441132 0.441132 0.450548 0.450548 0.450548 0.460189 0.460189 0.460189 0.467051 0.467051 0.467051 0.5 0.5 0.5 0.532949 0.532949 0.532949 0.539811 0.539811 0.539811 0.549452 0.549452 0.549452 0.558868 0.558868 0.558868 0.568006 0.568006 0.568006 0.576844 0.576844 0.576844 0.58539 0.58539 0.58539 0.593675 0.593675 0.593675 0.601744 0.601744 0.601744 0.609648 0.609648 0.609648 0.617438 0.617438 0.617438 0.625165 0.625165 0.625165 0.632874 0.632874 0.632874 0.640608 0.640608 0.640608 0.648401 0.648401 0.648401 0.656287 0.656287 0.656287 0.664294 0.664294 0.664294 0.672444 0.672444 0.672444 0.680759 0.680759 0.680759 0.689257 0.689257 0.689257 0.697953 0.697953 0.697953 0.706861 0.706861 0.706861 0.715992 0.715992 0.715992 0.725357 0.725357 0.725357 0.734965 0.734965 0.734965 0.744824 0.744824 0.744824 0.75494 0.75494 0.75494 0.765319 0.765319 0.765319 0.777716 0.777716 0.777716 0.794089 0.794089 0.794089 0.802889 0.802889 0.802889 0.812862 0.812862 0.812862 0.824009 0.824009 0.824009 0.836328 0.836328 0.836328 0.849822 0.849822 0.849822 0.864488 0.864488 0.864488 0.880328 0.880328 0.880328 0.897341 0.897341 0.897341 0.915527 0.915527 0.915527 0.934887 0.934887 0.934887 1 1 1 1
  arc A266 (-46.061, 67.6465) -> (-45.0662, 67.6711) centre (-45.7832, 76.5321) ccw
  spline S65 degree 3 poles (-41.581, 68.698) (-41.7174, 68.7702) (-41.8504, 68.8486) (-41.9788, 68.9341) (-42.017, 68.9595) (-42.0548, 68.9856) (-42.0921, 69.0122) (-42.1271, 69.0373) (-42.1618, 69.063) (-42.1959, 69.0892) (-42.2279, 69.1137) (-42.2595, 69.1388) (-42.2906, 69.1644) (-42.3196, 69.1882) (-42.3482, 69.2125) (-42.3764, 69.2373) (-42.4025, 69.2603) (-42.4282, 69.2837) (-42.4535, 69.3075) (-42.4767, 69.3294) (-42.4996, 69.3517) (-42.5222, 69.3744) (-42.5427, 69.3951) (-42.563, 69.4161) (-42.5828, 69.4375) (-42.6008, 69.4569) (-42.6184, 69.4765) (-42.6357, 69.4965) (-42.6513, 69.5143) (-42.6667, 69.5323) (-42.6813, 69.5508) (-42.6942, 69.567) (-42.7065, 69.5837) (-42.7199, 69.6) (-42.7447, 69.6304) (-42.7731, 69.6599) (-42.7863, 69.6955) (-42.7964, 69.7224) (-42.7977, 69.7529) (-42.8022, 69.7822) (-42.806, 69.8067) (-42.812, 69.8304) (-42.8179, 69.8542) (-42.8236, 69.8775) (-42.8292, 69.9008) (-42.8353, 69.924) (-42.8412, 69.9466) (-42.8476, 69.9691) (-42.8543, 69.9914) (-42.8608, 70.0132) (-42.8677, 70.0349) (-42.8749, 70.0565) (-42.8819, 70.0776) (-42.8893, 70.0985) (-42.8971, 70.1193) (-42.9046, 70.1396) (-42.9125, 70.1597) (-42.9207, 70.1797) (-42.9288, 70.1992) (-42.9371, 70.2186) (-42.9459, 70.2378) (-42.9544, 70.2566) (-42.9633, 70.2752) (-42.9725, 70.2936) (-42.9815, 70.3116) (-42.9909, 70.3294) (-43.0006, 70.347) (-43.0101, 70.3643) (-43.02, 70.3813) (-43.0302, 70.3982) (-43.0403, 70.4147) (-43.0506, 70.431) (-43.0614, 70.447) (-43.0719, 70.4628) (-43.0828, 70.4783) (-43.0941, 70.4936) (-43.1052, 70.5086) (-43.1166, 70.5234) (-43.1284, 70.5379) (-43.1401, 70.5522) (-43.1522, 70.5662) (-43.1646, 70.5798) (-43.1769, 70.5934) (-43.1896, 70.6066) (-43.2027, 70.6194) (-43.2157, 70.6322) (-43.2291, 70.6447) (-43.2429, 70.6567) (-43.2567, 70.6687) (-43.2709, 70.6803) (-43.2854, 70.6914) (-43.3001, 70.7025) (-43.3152, 70.7132) (-43.3306, 70.7233) (-43.3463, 70.7336) (-43.3624, 70.7433) (-43.3788, 70.7523) (-43.3955, 70.7615) (-43.4126, 70.7701) (-43.4301, 70.7779) (-43.448, 70.7859) (-43.4663, 70.7931) (-43.4849, 70.7994) (-43.5041, 70.806) (-43.5235, 70.8116) (-43.5433, 70.8162) (-43.5637, 70.821) (-43.5843, 70.8247) (-43.6051, 70.8273) (-43.6266, 70.83) (-43.6482, 70.8314) (-43.6699, 70.8317) (-43.6922, 70.8319) (-43.7145, 70.8308) (-43.7367, 70.8283) (-43.7594, 70.8258) (-43.782, 70.8218) (-43.8042, 70.8165) (-43.82, 70.8128) (-43.8357, 70.8085) (-43.8513, 70.8039) (-43.9263, 70.7821) (-43.9998, 70.7555) (-44.0746, 70.7334) (-44.1495, 70.7114) (-44.2257, 70.6939) (-44.3005, 70.6716) (-44.3161, 70.667) (-44.3316, 70.6621) (-44.3469, 70.6566) (-44.3684, 70.649) (-44.3895, 70.6401) (-44.41, 70.6299) (-44.43, 70.62) (-44.4493, 70.6088) (-44.468, 70.5965) (-44.486, 70.5846) (-44.5034, 70.5716) (-44.52, 70.5577) (-44.5361, 70.5443) (-44.5514, 70.5299) (-44.566, 70.5149) (-44.58, 70.5003) (-44.5933, 70.485) (-44.6059, 70.4691) (-44.6181, 70.4537) (-44.6295, 70.4377) (-44.6403, 70.4213) (-44.6507, 70.4053) (-44.6605, 70.3888) (-44.6695, 70.372) (-44.6784, 70.3555) (-44.6867, 70.3387) (-44.6943, 70.3215) (-44.7017, 70.3047) (-44.7086, 70.2875) (-44.7149, 70.2702) (-44.7211, 70.253) (-44.7268, 70.2355) (-44.7318, 70.2179) (-44.7369, 70.2004) (-44.7414, 70.1827) (-44.7455, 70.1649) (-44.7495, 70.147) (-44.753, 70.129) (-44.756, 70.1109) (-44.759, 70.0927) (-44.7615, 70.0744) (-44.7636, 70.0561) (-44.7657, 70.0375) (-44.7673, 70.0189) (-44.7685, 70.0002) (-44.7697, 69.9813) (-44.7704, 69.9623) (-44.7707, 69.9434) (-44.771, 69.9241) (-44.7709, 69.9047) (-44.7704, 69.8854) (-44.7698, 69.8658) (-44.7689, 69.8461) (-44.7675, 69.8264) (-44.7661, 69.8063) (-44.7643, 69.7863) (-44.7621, 69.7663) (-44.7599, 69.7458) (-44.7573, 69.7253) (-44.7543, 69.705) (-44.7512, 69.6841) (-44.7477, 69.6633) (-44.7439, 69.6425) (-44.74, 69.6212) (-44.7357, 69.6) (-44.731, 69.5789) (-44.7263, 69.5572) (-44.7211, 69.5357) (-44.7156, 69.5142) (-44.71, 69.4921) (-44.704, 69.4702) (-44.6976, 69.4483) (-44.6911, 69.4259) (-44.6843, 69.4035) (-44.677, 69.3813) (-44.6696, 69.3585) (-44.6616, 69.3359) (-44.6538, 69.3133) (-44.6458, 69.2901) (-44.638, 69.2669) (-44.6279, 69.2442) (-44.6158, 69.2172) (-44.6005, 69.1909) (-44.5943, 69.1628) (-44.5861, 69.1257) (-44.594, 69.0855) (-44.5984, 69.0465) (-44.6007, 69.0255) (-44.6021, 69.0049) (-44.6041, 68.9842) (-44.6063, 68.9608) (-44.6095, 68.9373) (-44.6129, 68.9139) (-44.6167, 68.8877) (-44.6208, 68.8617) (-44.6254, 68.8357) (-44.6305, 68.8069) (-44.6361, 68.7783) (-44.6421, 68.7497) (-44.6487, 68.7184) (-44.6559, 68.6873) (-44.6636, 68.6563) (-44.6719, 68.6225) (-44.6808, 68.5889) (-44.6903, 68.5555) (-44.7005, 68.5194) (-44.7114, 68.4835) (-44.7228, 68.4477) (-44.7351, 68.4093) (-44.748, 68.3712) (-44.7616, 68.3332) (-44.7761, 68.2926) (-44.7913, 68.2523) (-44.8071, 68.2123) (-44.824, 68.1696) (-44.8416, 68.1273) (-44.8599, 68.0852) (-44.9215, 67.9437) (-44.9907, 67.8057) (-45.0662, 67.6711) knots 0 0 0 0 0.065113 0.065113 0.065113 0.084473 0.084473 0.084473 0.102659 0.102659 0.102659 0.119672 0.119672 0.119672 0.135512 0.135512 0.135512 0.150178 0.150178 0.150178 0.163672 0.163672 0.163672 0.175991 0.175991 0.175991 0.187138 0.187138 0.187138 0.197111 0.197111 0.197111 0.205911 0.205911 0.205911 0.222284 0.222284 0.222284 0.234681 0.234681 0.234681 0.24506 0.24506 0.24506 0.255176 0.255176 0.255176 0.265035 0.265035 0.265035 0.274643 0.274643 0.274643 0.284008 0.284008 0.284008 0.293139 0.293139 0.293139 0.302047 0.302047 0.302047 0.310743 0.310743 0.310743 0.319241 0.319241 0.319241 0.327556 0.327556 0.327556 0.335706 0.335706 0.335706 0.343713 0.343713 0.343713 0.351599 0.351599 0.351599 0.359392 0.359392 0.359392 0.367126 0.367126 0.367126 0.374835 0.374835 0.374835 0.382562 0.382562 0.382562 0.390352 0.390352 0.390352 0.398256 0.398256 0.398256 0.406325 0.406325 0.406325 0.41461 0.41461 0.41461 0.423156 0.423156 0.423156 0.431994 0.431994 0.431994 0.441132 0.441132 0.441132 0.450548 0.450548 0.450548 0.460189 0.460189 0.460189 0.467051 0.467051 0.467051 0.5 0.5 0.5 0.532949 0.532949 0.532949 0.539811 0.539811 0.539811 0.549452 0.549452 0.549452 0.558868 0.558868 0.558868 0.568006 0.568006 0.568006 0.576844 0.576844 0.576844 0.58539 0.58539 0.58539 0.593675 0.593675 0.593675 0.601744 0.601744 0.601744 0.609648 0.609648 0.609648 0.617438 0.617438 0.617438 0.625165 0.625165 0.625165 0.632874 0.632874 0.632874 0.640608 0.640608 0.640608 0.648401 0.648401 0.648401 0.656287 0.656287 0.656287 0.664294 0.664294 0.664294 0.672444 0.672444 0.672444 0.680759 0.680759 0.680759 0.689257 0.689257 0.689257 0.697953 0.697953 0.697953 0.706861 0.706861 0.706861 0.715992 0.715992 0.715992 0.725357 0.725357 0.725357 0.734965 0.734965 0.734965 0.744824 0.744824 0.744824 0.75494 0.75494 0.75494 0.765319 0.765319 0.765319 0.777716 0.777716 0.777716 0.794089 0.794089 0.794089 0.802889 0.802889 0.802889 0.812862 0.812862 0.812862 0.824009 0.824009 0.824009 0.836328 0.836328 0.836328 0.849822 0.849822 0.849822 0.864488 0.864488 0.864488 0.880328 0.880328 0.880328 0.897341 0.897341 0.897341 0.915527 0.915527 0.915527 0.934887 0.934887 0.934887 1 1 1 1
  arc A267 (-41.581, 68.698) -> (-40.7317, 69.2168) centre (-45.7832, 76.5321) ccw